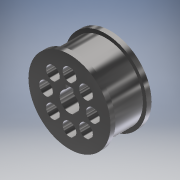
# Autodesk Inventor part: 24 Teeth HTD5M Pulley Steel
Saved by Autodesk Inventor 2019.4 (Build 234330000, 330)
## iProperties
Created: 2019-12-31
Part Number: 24 Teeth HTD5M Pulley Steel
Material: Stainless Steel
Document SubType Name: Modeling
Designer: Mark
Mass: 135.897 g
Surface Area: 94.8611 cm^2
Volume: 16.9871 cm^3
Density: 8 g/cm^3
Appearance: Semi-Polished
Author: Mark
Autodesk Inventor part; units mm, degrees
ref_plane "YZ Plane" through (0, 0, 0) normal (1, 0, 0) x (0, 1, 0)
ref_plane "XZ Plane" through (0, 0, 0) normal (0, 1, 0) x (-1, 0, 0)
ref_plane "XY Plane" through (0, 0, 0) normal (0, 0, 1) x (1, 0, 0)
sketch "Sketch1" plane through (0, 0, 0) normal (0, 0, 1) x (1, 0, 0)
  circle A0 centre (0, 0) radius 21
  dimension "d0" = 42
  constraints: 1 centre point, 1 coincident
  measures "d0" diameter of A0
extrude "Extrusion1" add sketch "Sketch1" along normal blind 2.5
sketch "Sketch2" plane through (0, 0, 2.5) normal (0, 0, 1) x (1, 0, 0)
  circle A0 centre (0, 0) radius 19.1
  dimension "d3" = 38.2
  constraints: 1 centre point, 1 coincident
  measures "d3" diameter of A0
extrude "Extrusion2" add sketch "Sketch2" along normal blind 16
sketch "Sketch3" plane through (0, 0, 18.5) normal (0, 0, 1) x (1, 0, 0)
  circle A0 centre (0, 0) radius 21
  dimension "d6" = 42
  constraints: 1 centre point, 1 coincident
  measures "d6" diameter of A0
extrude "Extrusion3" add sketch "Sketch3" along normal blind 2.5
sketch "Sketch4" plane through (0, 0, 21) normal (0, 0, 1) x (1, 0, 0)
  circle A0 centre (0, 0) radius 5
  line L0 (-2, 3.2) -> (2, 3.2)
  line L1 (2, 3.2) -> (2, 6.8)
  line L2 (2, 6.8) -> (-2, 6.8)
  line L3 (-2, 6.8) -> (-2, 3.2)
  line L4 (-2, 3.2) -> (2, 6.8) construction
  line L5 (2, 3.2) -> (-2, 6.8) construction
  point P0 (0, 5)
  dimension "d9" = 10
  dimension "d10" = 4
  dimension "d11" = 3.6
  constraints: 12 end point, 2 midpoint, 2 parallel, 1 coincident, 1 horizontal, 1 perpendicular, 1 vertical alignment, 2 other
  measures "d10" distance of L2.end L1.end
  measures "d11" distance of L1.end L0.end
extrude "Extrusion4" cut sketch "Sketch4" against normal blind 21
sketch "Sketch5" plane through (0, 0, 21) normal (0, 0, 1) x (1, 0, 0)
  circle A0 centre (0, -12) radius 3.5
  arc A1 (-2, 4.5826) -> (2, 4.5826) centre (0, 0) ccw projected
  line L0 (0, 0) -> (0, -12)
  line L1 (0, 0) -> (12, 0) construction
  circle A2 centre (8.4853, -8.4853) radius 3.5
  circle A3 centre (12, 0) radius 3.5
  circle A4 centre (8.4853, 8.4853) radius 3.5
  circle A5 centre (0, 12) radius 3.5
  circle A6 centre (-8.4853, 8.4853) radius 3.5
  circle A7 centre (-12, 0) radius 3.5
  circle A8 centre (-8.4853, -8.4853) radius 3.5
  dimension "d14" = 7
  dimension "d15" = 12
  dimension "d16" = 90
  dimension "d19" = 360
  constraints: 8 centre point, 4 end point, 1 coincident, 1 horizontal, 1 perpendicular, 17 other
  measures "d14" diameter of A0
  measures "d15" distance of L0.start A0.centre
  measures "d16" angle of L0 L1
extrude "Extrusion5" cut sketch "Sketch5" against normal blind 21
body "Solid1"
